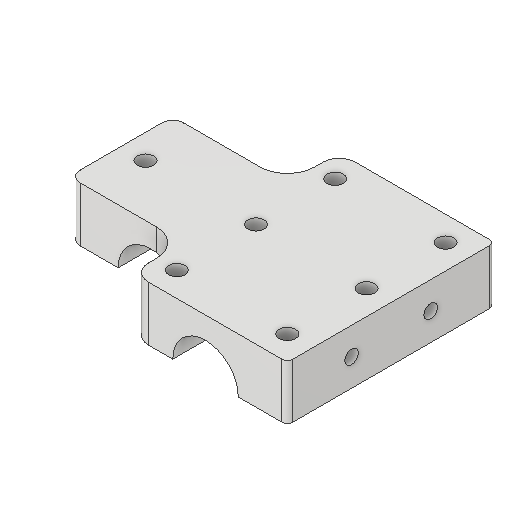
# Autodesk Inventor part: 3DP_PLA_X_axis_carriage_half
Saved by Autodesk Inventor 2026.1 (Build 301233000, 233)
## iProperties
Created: 2018-07-08
Part Number: 3DP_PLA_X_axis_carriage_half
Material: ABS Plastic
Document SubType Name: Modeling
Designer: Andrzej
Density: 1.06 g/cm^3
Appearance: Smooth - White
Author: Andrzej
Autodesk Inventor part; units mm, degrees
ref_plane "YZ Plane" through (0, 0, 0) normal (1, 0, 0) x (0, 1, 0)
ref_plane "XZ Plane" through (0, 0, 0) normal (0, 1, 0) x (-1, 0, 0)
ref_plane "XY Plane" through (0, 0, 0) normal (0, 0, 1) x (1, 0, 0)
sketch "Sketch1" plane through (0, 0, 0) normal (0, 0, 1) x (1, 0, 0)
  circle A0 centre (9.0035, 0) radius 6
  circle A1 centre (-10.4965, 0) radius 6
  line L0 (-16.4965, 0) -> (-25.4965, 0)
  line L1 (-25.4965, 0) -> (-25.4965, 10)
  line L2 (-25.4965, 10) -> (24.0035, 10)
  line L3 (24.0035, 10) -> (24.0035, 0)
  line L4 (24.0035, 0) -> (15.0035, 0)
  line L5 (-4.4965, 0) -> (3.0035, 0)
  point P0 (0, 0)
  dimension "d4" = 12
  dimension "d5" = 12
  dimension "d6" = 19.5
  dimension "d7" = 0
  dimension "d8" = 0
  dimension "d9" = 9
  dimension "d10" = 9
  dimension "d11" = 10
  dimension "d12" = 0
  constraints: 12 end point, 4 point on circle, 3 perpendicular, 2 centre point, 2 horizontal, 2 point on line, 1 other
  measures "d4" diameter of A0
  measures "d5" diameter of A1
  measures "d6" distance of A0.centre A1.centre
  measures "d7" distance from line of point (0, 0) L0
  measures "d8" distance from line of point (0, 0) L4
  measures "d9" distance from line of L1 L0.start
  measures "d10" distance from line of L4.end L3
  measures "d11" distance from line of L2 A1.centre
  measures "d12" distance from line of point (0, 0) L5
extrude "Extrusion1" add sketch "Sketch1" along normal blind 38 contours A0 L5 A1 L0 L1 L2 L3 L4
sketch "Sketch2" plane through (-4.4965, 0, 0) normal (0, -1, 0) x (1, 0, 0)
  line L0 (-21, 0) -> (-12, 0) projected
  line L1 (-12, 0) -> (-12, 38) projected
  line L2 (-21, 38) -> (-12, 38) projected
  line L3 (-21, 0) -> (-21, 38) projected
  line L4 (0, 0) -> (7.5, 0) projected
  line L5 (7.5, 0) -> (7.5, 38) projected
  line L6 (0, 38) -> (7.5, 38) projected
  line L7 (0, 0) -> (0, 38) projected
  line L8 (19.5, 0) -> (28.5, 0) projected
  line L9 (28.5, 0) -> (28.5, 38) projected
  line L10 (19.5, 38) -> (28.5, 38) projected
  line L11 (19.5, 0) -> (19.5, 38) projected
  line L12 (-21, 0) -> (-12, 0) projected
  line L13 (-21, 0) -> (0, 0)
  line L14 (-21, 9.5) -> (0, 9.5)
  line L15 (-21, 28.5) -> (0, 28.5)
  line L16 (0, 0) -> (0, 38) projected
  line L17 (-12, 38) -> (0, 38) projected
  line L18 (-21, 38) -> (0, 38)
  point P0 (4.4965, 0)
  dimension "d17" = 19
  dimension "d18" = 9.5
  constraints: 8 end point, 4 point on line, 2 collinear, 2 perpendicular
  measures "d17" distance between parallel lines of L15 L14
  measures "d18" distance between parallel lines of L0 L14
extrude "Extrusion2" cut sketch "Sketch2" against normal through all contours L3 L14 L1 L0 | L1 L14 L7 L13 | L3 L2 L1 L15 | L1 L17 L7 L15
fillet "Fillet1" radius 5 2 edges at (-4.4965, 5, 28.5) (-4.4965, 5, 9.5)
fillet "Fillet2" radius 3 2 edges at (-4.4965, 5, 0) (-4.4965, 5, 38)
fillet "Fillet2" radius 1 2 edges at (24.0035, 5, 38) (24.0035, 5, 0)
fillet "Fillet2" radius 2 2 edges at (-25.4965, 5, 9.5) (-25.4965, 5, 28.5)
sketch "Sketch3" plane through (3.0035, 0, 0) normal (0, -1, 0) x (1, 0, 0)
  arc A0 (-28.5, 11.5) -> (-26.5, 9.5) centre (-26.5, 11.5) ccw projected
  line L0 (-26.5, 9.5) -> (-19.5, 9.5) projected
  line L1 (-19.5, 9.5) -> (-19.5, 28.5) projected
  line L2 (-19.5, 28.5) -> (-26.5, 28.5) projected
  arc A1 (-26.5, 28.5) -> (-28.5, 26.5) centre (-26.5, 26.5) ccw projected
  line L3 (-28.5, 11.5) -> (-28.5, 26.5) projected
  arc A2 (-4.5, 38) -> (-7.5, 35) centre (-4.5, 35) ccw projected
  line L4 (-7.5, 33.5) -> (-7.5, 35) projected
  line L5 (-7.5, 4.5) -> (-7.5, 33.5) projected
  line L6 (-7.5, 3) -> (-7.5, 4.5) projected
  arc A3 (-7.5, 3) -> (-4.5, 0) centre (-4.5, 3) ccw projected
  line L7 (-4.5, 0) -> (0, 0) projected
  line L8 (0, 0) -> (0, 38) projected
  line L9 (-4.5, 38) -> (0, 38) projected
  arc A4 (21, 37) -> (20, 38) centre (20, 37) ccw projected
  line L10 (12, 38) -> (20, 38) projected
  line L11 (12, 0) -> (12, 38) projected
  line L12 (12, 0) -> (20, 0) projected
  arc A5 (20, 0) -> (21, 1) centre (20, 1) ccw projected
  line L13 (21, 1) -> (21, 37) projected
  point P0 (-3.0035, 0)
  point P1 (-3.75, 4.5)
  point P2 (-3.75, 19)
  point P3 (-3.75, 33.5)
  point P4 (16.5, 4.5)
  point P5 (16.5, 19)
  point P6 (16.5, 33.5)
  point P7 (-24, 19)
  dimension "d23" = 7.5
  dimension "d24" = 3.75
  dimension "d25" = 9
  dimension "d26" = 4.5
  dimension "d27" = 9
  dimension "d28" = 4.5
  dimension "d29" = 19
  dimension "d30" = 9.5
  dimension "d31" = 4.5
  dimension "d32" = 4.5
  constraints: 4 horizontal alignment, 4 vertical alignment
  measures "d23" distance between parallel lines of L5 L8
  measures "d24" distance from line of L8 point (-3.75, 4.5)
  measures "d25" distance between parallel lines of L13 L11
  measures "d26" distance from line of L13 point (16.5, 4.5)
  measures "d27" distance between parallel lines of L1 L3
  measures "d28" distance from line of L3 point (-24, 19)
  measures "d29" distance between parallel lines of L2 L0
  measures "d30" distance from line of L0 point (-24, 19)
  measures "d31" distance from line of L7 point (-3.75, 4.5)
  measures "d32" distance from line of L9 point (-3.75, 33.5)
hole "Hole1" at (-0.7465, 0, 4.5) at (-0.7465, 0, 19) at (-0.7465, 0, 33.5) at (19.5035, 0, 4.5) at (19.5035, 0, 19) at (19.5035, 0, 33.5) at (-20.9965, 0, 19) direction (0, 1, 0) diameter 3 end through all
sketch "Sketch4" plane through (24.0035, 0, 1) normal (1, 0, 0) x (0, 0, -1)
  line L0 (-16.5, 10) -> (-16.5, 0) projected
  line L1 (-19.5, 10) -> (-19.5, 0) projected
  line L2 (-31, 10) -> (-31, 0) projected
  line L3 (-5, 10) -> (-5, 0) projected
  line L4 (0, 10) -> (0, 0) projected
  line L5 (0, 10) -> (-36, 10) projected
  line L6 (-36, 0) -> (-36, 10) projected
  line L7 (0, 0) -> (-36, 0) projected
  point P0 (1, 0)
  point P1 (-25.25, 5)
  point P2 (-10.75, 5)
  dimension "d41" = 11.5
  dimension "d42" = 11.5
  dimension "d43" = 5.75
  dimension "d44" = 5.75
  dimension "d45" = 10
  dimension "d46" = 5
  constraints: 1 horizontal alignment
  measures "d41" distance between parallel lines of L1 L2
  measures "d42" distance between parallel lines of L3 L0
  measures "d43" distance from line of L2 point (-25.25, 5)
  measures "d44" distance from line of L0 point (-10.75, 5)
  measures "d46" vertical distance of L5 point (-10.75, 5)
hole "Hole2" at (24.0035, 5, 26.25) at (24.0035, 5, 11.75) direction (-1, 0, 0) diameter 2.5 depth 8 tip angle 118
equation "\"d24\" = 0.5 * d23"
equation "\"d26\" = 0.5 * d25"
equation "\"d28\" = 0.5 * d27"
equation "\"d30\" = 0.5 * d29"
equation "\"d32\" = d31"
equation "\"d43\" = 0.5 * d41"
equation "\"d44\" = 0.5 * d42"
equation "\"d46\" = 0.5 * d45"
body "Solid1"
